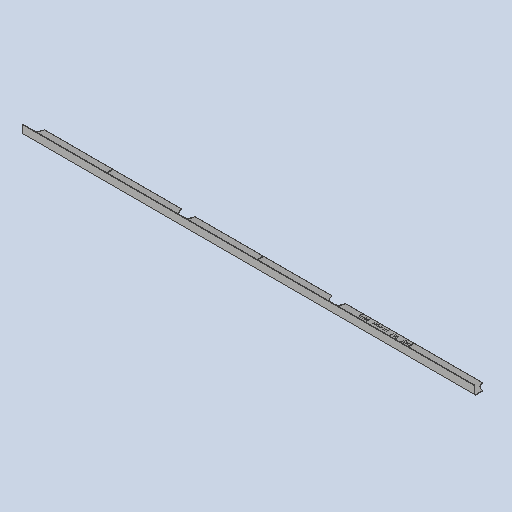
# Autodesk Inventor part: MSC 057 stringer belly
Saved by Autodesk Inventor 2024.2 (Build 282272000, 272)
## iProperties
Created: 2024-04-28
Part Number: MSC 057 stringer belly
Material: Stainless Steel
Document SubType Name: Sheet Metal
Designer: pokla
Density: 8 g/cm^3
Flat Pattern Width: 7.6202 cm
Flat Pattern Length: 150 cm
Flat Pattern Area: 1143.03 cm^2
Sheet Metal Rule: AISI304 2mm Die16
Sheet Metal Width: 76,202 mm
Sheet Metal Length: 1500,000 mm
Sheet Metal Area: 114302,986 mm^2
Appearance: Default
Stock Number: МОО 057 стрингер борт живот
Author: admin
Autodesk Inventor part; units mm, degrees
ref_plane "YZ Plane" through (0, 0, 0) normal (1, 0, 0) x (0, 1, 0)
ref_plane "XZ Plane" through (0, 0, 0) normal (0, 1, 0) x (-1, 0, 0)
ref_plane "XY Plane" through (0, 0, 0) normal (0, 0, 1) x (1, 0, 0)
sketch "Sketch1" plane through (0, 0, 0) normal (0, 0, 1) x (1, 0, 0)
  line L0 (-750, 50) -> (750, 50)
  line L1 (750, 50) -> (750, 0)
  line L2 (750, 0) -> (-750, 0)
  line L3 (-750, 0) -> (-750, 50)
  point P0 (0, 0)
  point P1 (0, 0)
  dimension "d0" = 1500
  dimension "d1" = 50
  measures "d0" distance of L1.end L2.end
  measures "d1" distance of L0.end L1.end
extrude "Plate1" add sketch "Sketch1" along normal blind 2
sketch "Sketch2" plane through (750, 2, 0) normal (0, -1, 0) x (1, 0, 0)
  line L0 (-1500, 0) -> (0, 0)
  line L1 (0, 0) -> (0, 30)
  line L2 (0, 30) -> (-1500, 30)
  line L3 (-1500, 30) -> (-1500, 0)
  constraints: 6 end point, 1 horizontal, 1 perpendicular, 1 vertical
edge flange "Flange1" height 30 angle 90 thickness 2 bend radius 2.75 thickness toward (0, -1, 0) relief round relief width 2 relief depth 1 edges at (0, 0, 2) wall of the first edge with corners at (-750, 2, 0) (750, 2, 0) (750, 2, 30) (-750, 2, 30)
bend "Bend1"
corner "Corner1"
sketch "Sketch5" plane through (0, 0, 0) normal (0, 0, -1) x (-1, 0, 0)
  line L0 (750, 50) -> (-750, 50) projected
  line L1 (-1, 30) -> (-1, 50)
  line L2 (750, 0) -> (-750, 0) projected
  line L3 (-1, 30) -> (1, 30)
  line L4 (1, 30) -> (1, 50)
  point P0 (0, 0)
  point P1 (0, 30)
  point P2 (0, 0)
  dimension "d27" = 2
  dimension "d28" = 30
  constraints: 6 end point, 2 midpoint, 2 point on line, 1 horizontal, 1 parallel, 1 perpendicular, 1 vertical alignment
  measures "d27" distance of L1.start L3.end
  measures "d28" distance of point (0, 0) point (0, 30)
extrude "Extrusion1" cut sketch "Sketch5" against normal through all
pattern_linear "Rectangular Pattern1" count 3 spacing 500 along (1, 0, 0) of "Extrusion1" first direction both ways yes
sketch "Sketch6" plane through (0, 0, 0) normal (0, 0, -1) x (-1, 0, 0)
  line L0 (-750, 50) -> (-750, 4.75) projected
  circle A0 centre (-750, 50) radius 22.5
  line L1 (-750, 50) -> (750, 50) projected
  line L2 (-1, 50) -> (-1, 30) projected
  line L3 (-499, 50) -> (-499, 30) projected
  line L4 (-1, 30) -> (-499, 30) construction
  circle A1 centre (-250, 50) radius 22.5
  point P0 (0, 0)
  point P1 (-727.5, 50)
  point P2 (-750, 27.5)
  point P3 (-250, 30)
  dimension "d24" = 45
  constraints: 2 centre point, 2 end point, 1 equal radius, 1 midpoint, 1 perpendicular, 1 point on line, 1 vertical alignment
  measures "d24" diameter of A0
extrude "Extrusion2" cut sketch "Sketch6" along normal mid plane 30 contours L1 A0 L0 | A1 L1 | L1 A1 picked at (-748.3311, 35.188)
mirror "Mirror1" about plane through (0, 0, 0) normal (1, 0, 0) of "Extrusion2"
sketch "Sketch7" plane through (0, 0, 2) normal (0, 0, 1) x (1, 0, 0)
  line L0 (494, 45) -> (494, 33) construction
  line L1 (494, 33) -> (294, 33) construction
  line L2 (294, 33) -> (294, 45) construction
  line L3 (294, 45) -> (494, 45) construction
  line L4 (272.5, 50) -> (499, 50) projected
  point P0 (0, 0)
  dimension "d29" = 200
  dimension "d30" = 12
  dimension "d31" = 5
  dimension "d32" = 5
  constraints: 2 other
  measures "d29" distance of L0.end L2.start
  measures "d30" distance of L2.start L2.end
  measures "d31" distance between parallel lines of L4 L3
  measures "d32" distance from line of L4.end L0
mark "Mark1"
equation "\"d28\" = Стрингер_глубина_паза"
equation "\"d1\" = Стрингер_7"
equation "\"d27\" = d18"
equation "\"d2\" = Thickness"
equation "\"d3\" = BendReliefWidth"
equation "\"d4\" = BendReliefDepth"
equation "\"d5\" = MinimumRemnant"
equation "\"d6\" = TransitionRadius"
equation "\"d9\" = BendRadius"
equation "\"d10\" = CornerReliefSize"
equation "\"d11\" = GapSize"
equation "\"d12\" = JacobiRadiusSize"
equation "\"GapSize\" = Thickness"
equation "\"MinimumRemnant\" = 2 * Thickness"
equation "\"BendReliefDepth\" = 0.5 * Thickness"
equation "\"BendReliefWidth\" = Thickness"
equation "\"CornerReliefSize\" = 4 * Thickness"
equation "\"JacobiRadiusSize\" = BendRadius"
equation "\"TransitionRadius\" = BendRadius"
equation "\"d18\" = Thickness"
equation "\"Стрингер_7\" = 50"
equation "\"Thickness\" = 2"
equation "\"BendRadius\" = 2.75"
equation "\"Стрингер_глубина_паза\" = 30"
body "Solid1"
